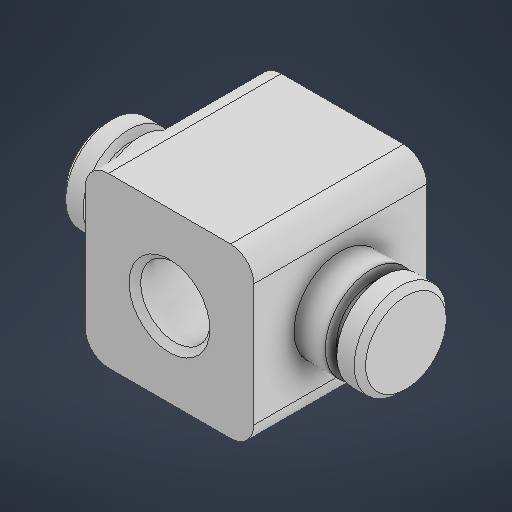
# Autodesk Inventor part: Tee
Saved by Autodesk Inventor 2025.4 (Build 294407000, 407)
## iProperties
Created: 2026-05-27
Part Number: Tee
Material: Generic
Document SubType Name: Modeling
Designer: VuQuan
Density: 1 g/cm^3
Appearance: Default
Author: VuQuan
Autodesk Inventor part; units mm, degrees
ref_plane "YZ Plane" through (0, 0, 0) normal (1, 0, 0) x (0, 1, 0)
ref_plane "XZ Plane" through (0, 0, 0) normal (0, 1, 0) x (-1, 0, 0)
ref_plane "XY Plane" through (0, 0, 0) normal (0, 0, 1) x (1, 0, 0)
sketch "Sketch1" plane through (0, 0, 0) normal (0, 0, 1) x (1, 0, 0)
  line L0 (-5.3, 7.3) -> (5.3, 7.3)
  line L1 (7.3, 5.3) -> (7.3, -5.3)
  line L2 (5.3, -7.3) -> (-5.3, -7.3)
  line L3 (-7.3, -5.3) -> (-7.3, 5.3)
  arc A0 (-5.3, 7.3) -> (-7.3, 5.3) centre (-5.3, 5.3) ccw
  arc A1 (7.3, 5.3) -> (5.3, 7.3) centre (5.3, 5.3) ccw
  arc A2 (5.3, -7.3) -> (7.3, -5.3) centre (5.3, -5.3) ccw
  arc A3 (-7.3, -5.3) -> (-5.3, -7.3) centre (-5.3, -5.3) ccw
  line L4 (-7.3, 4) -> (-10, 4)
  line L5 (-10, 4) -> (-10, 3)
  line L6 (-10, 3) -> (-11, 3)
  line L7 (-11, 3) -> (-11, 4)
  line L8 (-11, 4) -> (-13, 4)
  line L9 (-13, 4) -> (-13, 0)
  line L10 (-13, 0) -> (-7.3, 0)
  circle A4 centre (0, 0) radius 3
  point P0 (0, 7.3)
  point P1 (7.3, 0)
  dimension "d0" = 14.6
  dimension "d1" = 2
  dimension "d3" = 8
  dimension "d4" = 6
  dimension "d5" = 2
  dimension "d6" = 1
  dimension "d7" = 13
  dimension "d11" = 6
  constraints: 22 end point, 8 point on circle, 8 tangent, 6 perpendicular, 5 centre point, 3 equal radius, 3 horizontal, 3 midpoint, 3 point on line, 2 parallel, 1 coincident, 1 horizontal alignment, 1 vertical alignment
  measures "d0" distance between parallel lines of L1 L3
  measures "d1" radius of A0
  measures "d3" diameter of L8 L10
  measures "d4" diameter of L6 L10
  measures "d5" distance between parallel lines of L7 L9
  measures "d6" distance between parallel lines of L5 L7
  measures "d7" distance from line of point (0, 0) L9
  measures "d11" diameter of A4
extrude "Extrusion1" add sketch "Sketch1" along normal mid plane 15 contours L0 A1 L1 A2 L2 A3 L3 A0
revolve "Revolution1" add sketch "Sketch1" angle 360 about axis through (-13, 0, 0) along (1, 0, 0) contours L3 L10 L9 L8 L7 L6 L5 L4
mirror "Mirror1" about plane through (0, 0, 0) normal (1, 0, 0) of "Revolution1"
chamfer "Chamfer1" distance 0.5 angle 45 4 edges at (13, -4, 0) (-13, -4, 0) (-3, 0, 7.5) (-3, 0, -7.5)
body "Solid1"
